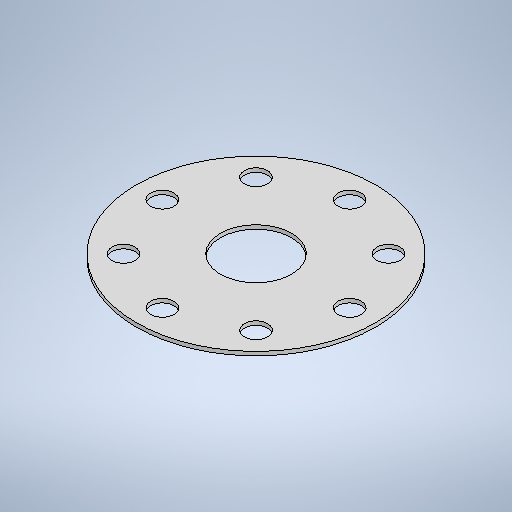
# Autodesk Inventor part: MSC 922 plug 76 hole
Saved by Autodesk Inventor 2025.1 (Build 291241020, 241B)
## iProperties
Created: 2024-11-20
Part Number: MSC 922 plug 76 hole
Material: Stainless Steel
Document SubType Name: Sheet Metal
Designer: user
Mass: 280.619 g
Surface Area: 364.406 cm^2
Volume: 35.0774 cm^3
Density: 8 g/cm^3
Flat Pattern Width: 18.5 cm
Flat Pattern Length: 18.5 cm
Flat Pattern Area: 342.25 cm^2
Sheet Metal Rule: AISI304 3mm Die 32
Sheet Metal Width: 185.000 mm
Sheet Metal Length: 185.000 mm
Sheet Metal Area: 34225.000 mm^2
Appearance: Default
Author: user
Autodesk Inventor part; units mm, degrees
ref_plane "YZ Plane" through (0, 0, 0) normal (1, 0, 0) x (0, 1, 0)
ref_plane "XZ Plane" through (0, 0, 0) normal (0, 1, 0) x (-1, 0, 0)
ref_plane "XY Plane" through (0, 0, 0) normal (0, 0, 1) x (1, 0, 0)
sketch "Sketch1" plane through (0, 0, 0) normal (0, 0, 1) x (1, 0, 0)
  circle A0 centre (0, 0) radius 92.5
  dimension "d22" = 185
  measures "d22" diameter of A0
extrude "Plate1" add sketch "Sketch1" along normal blind 3
sketch "Sketch5" plane through (0, 0, 3) normal (0, 0, 1) x (1, 0, 0)
  circle A0 centre (0, 0) radius 92.5 projected
  circle A1 centre (0, 72.5) radius 9
  circle A2 centre (0, 0) radius 72.5 construction
  dimension "d23" = 18
  dimension "d30" = 20
  constraints: 2 vertical alignment, 1 centre point, 1 coincident, 2 other
  measures "d23" diameter of A1
extrude "Cut1" cut sketch "Sketch5" against normal blind 3 contours A1
pattern_circular "Circular Pattern1" count 8 over 360 about axis through (0, 0, 0) along (0, 0, 1) of "Cut1"
sketch "Sketch6" plane through (0, 0, 0) normal (0, 0, -1) x (-1, 0, 0)
  circle A0 centre (0, 0) radius 27.5
  dimension "d31" = 55
  constraints: 1 centre point, 1 coincident
  measures "d31" diameter of A0
extrude "Cut2" cut sketch "Sketch6" against normal blind 3
equation "\"d25\" = Thickness"
equation "\"d32\" = Thickness"
equation "\"d2\" = Thickness"
equation "\"BendReliefWidth\" = Thickness"
equation "\"BendReliefDepth\" = 0.5 * Thickness"
equation "\"CornerReliefSize\" = 4 * Thickness"
equation "\"MinimumRemnant\" = 2 * Thickness"
equation "\"TransitionRadius\" = BendRadius"
equation "\"JacobiRadiusSize\" = BendRadius"
equation "\"GapSize\" = Thickness"
equation "\"Thickness\" = 3"
equation "\"BendRadius\" = 5"
body "Solid1"
